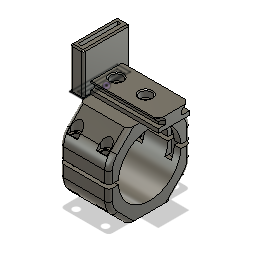
OBS-D-003 v10 (Autodesk Fusion 360 design; units mm, degrees)
Autodesk Fusion 360 part; units mm, degrees
sketch "Skizze1" plane through (0, 0, 0) normal (1, 0, 0) x (0, 0, -1)
  line L0 (-8, 5.2) -> (-6.05, 3.25)
  line L1 (-6.05, 3.25) -> (-6.05, 2)
  line L2 (6.05, 2) -> (6.05, 3.25)
  line L3 (6.05, 3.25) -> (8, 5.2)
  line L4 (8, 5.2) -> (8, 6.5)
  line L5 (8, 6.5) -> (-8, 6.5)
  line L6 (-8, 6.5) -> (-8, 5.2)
  line L7 (-6.05, 2) -> (-8, 2)
  line L8 (-8, 2) -> (-8, 0)
  line L9 (-8, 0) -> (8, 0)
  line L10 (8, 0) -> (8, 2)
  line L11 (8, 2) -> (6.05, 2)
  line L12 (0, 6.5) -> (0, 0) construction
  dimension "d5" = 16
  dimension "d6" = 1.3
  dimension "d8" = 2
  dimension "d26" = 12.1
  dimension "d27" = 4.5
  dimension "d28" = 135
  constraint vertical L1
  constraint perpendicular L2 L5
  constraint perpendicular L5 L6
  constraint vertical L4
  constraint perpendicular L1 L7
  constraint perpendicular L7 L8
  constraint perpendicular L8 L9
  constraint perpendicular L7 L10
  constraint perpendicular L2 L11
  constraint collinear L4 L10
  constraint collinear L6 L8
  constraint midpoint L5 L12.start
  constraint midpoint L9 L12.end
  constraint symmetric L0.start L3.end L12
  constraint symmetric L0.end L2.end L12
  constraint midpoint L12.end L9
  constraint collinear L7 L11
  measures "d5" distance of L4.end L5.end
  measures "d6" distance of L0.start L5.end
  measures "d8" distance of L7 L9
  measures "d26" distance of L1 L2
  measures "d27" distance of L5 L7
  measures "d28" angle of L0 L6
extrude "Extrusion1" add sketch "Skizze1" along normal blind 34.4 makes body 1
sketch "Skizze7" plane through (0, 0, 0) normal (0, 1, 0) x (1, 0, 0)
  line L0 (0, -12) -> (-6.6, -12)
  line L1 (-6.6, -12) -> (-6.6, 12)
  line L2 (-6.6, 12) -> (0, 12)
  line L3 (0, 12) -> (0, -12)
  line L4 (-0.8, -10) -> (-4.6, -10)
  line L5 (-4.6, -10) -> (-4.6, 10)
  line L6 (-4.6, 10) -> (-0.8, 10)
  line L7 (-0.8, 10) -> (-0.8, -10)
  line L8 (0, 0) -> (-0.8, 0) construction
  line L9 (-2.7, -10) -> (-2.7, 10)
  dimension "d82" = 24
  dimension "d83" = 0.8
  dimension "d84" = 2
  dimension "d85" = 3.8
  dimension "d86" = 20
  constraint horizontal L0
  constraint vertical L1
  constraint horizontal L2
  constraint vertical L3
  constraint midpoint L8.start L3
  constraint horizontal L4
  constraint vertical L5
  constraint horizontal L6
  constraint vertical L7
  constraint coincident L8.start origin
  constraint midpoint L7 L8.end
  constraint horizontal L8
  constraint midpoint L4 L9.start
  constraint midpoint L6 L9.end
  measures "d82" distance of L0.start L2.end
  measures "d83" distance of L3 L7
  measures "d84" distance of L1 L5
  measures "d85" distance of L5 L7
  measures "d86" distance of L4.end L5.end
extrude "Extrusion17" add sketch "Skizze7" along normal blind 21.2 bodies 1
extrude "Extrusion18" add sketch "Skizze7" along normal blind 9.7 contours L4 L6 L7 L9 | L4 L5 L6 L9 bodies 1
extrude "Extrusion19" add sketch "Skizze7" against normal blind 1.5 from surface at 21.2 contours L4 L6 L7 L9 bodies 1
sketch "Skizze3" plane through (0, 0, 0) normal (1, 0, 0) x (0, 0, -1)
  circle A0 centre (-2.9687, -21) radius 16
  line L0 (18, -20) -> (18, 0)
  line L1 (18, 0) -> (-23.9374, 0)
  line L2 (-23.9374, 0) -> (-23.9374, -20)
  line L3 (13, -20) -> (-18.9374, -20) construction
  line L4 (13, -20) -> (18, -20)
  line L5 (-18.9374, -20) -> (-23.9374, -20)
  line L6 (13, -22) -> (-18.9374, -22) construction
  line L7 (13, -22) -> (18, -22)
  line L8 (18, -22) -> (18, -42)
  line L9 (18, -42) -> (-23.9374, -42)
  line L10 (-23.9374, -42) -> (-23.9374, -22)
  line L11 (-23.9374, -22) -> (-18.9374, -22)
  line L12 (-2.9687, -21) -> (-2.9687, -5) construction
  line L13 (-2.9687, -37) -> (-2.9687, -21) construction
  dimension "d29" = 32
  dimension "d30" = 5
  dimension "d31" = 5
  dimension "d32" = 18
  dimension "d33" = 1
  dimension "d34" = 1
  dimension "d35" = 5
  dimension "d37" = 5
  constraint coincident A0 L3.start
  constraint coincident A0 L3.end
  constraint horizontal L3
  constraint horizontal L4
  constraint horizontal L5
  constraint vertical L0
  constraint coincident A0 L6.start
  constraint coincident A0 L6.end
  constraint horizontal L6
  constraint perpendicular L0 L7
  constraint perpendicular L10 L11
  constraint coincident A0.centre L12.start
  constraint coincident A0 L12.end
  constraint vertical L12
  constraint horizontal L1
  constraint vertical L2
  constraint vertical L8
  constraint horizontal L9
  constraint vertical L10
  constraint collinear L2 L10
  constraint collinear L0 L8
  constraint coincident A0 L13.start
  constraint perpendicular L6 L13
  constraint coincident origin L1
  measures "d29" diameter of A0
  measures "d30" distance of L0.start L3.start
  measures "d31" distance of L2.end L3.end
  measures "d32" distance of origin L0
  measures "d33" distance of A0.centre L3
  measures "d34" distance of A0.centre L6
  measures "d35" vertical distance of origin L12.end
  measures "d37" distance of L9 L13.start
extrude "Extrusion6" add sketch "Skizze3" along normal blind 25 separate body contours A0 L0 L1 L2 L4 L5 | A0 L7 L8 L9 L10 L11 makes body 2 at (8.3333, -6.3069, 9.3023) makes body 3 at (16.6667, -33.2963, -7.2686)
chamfer "Fase1" distance 10 angle 45 3 edges at (12.5, 0, 23.9374) (12.5, -42, -18) (12.5, -42, 23.9374) on bodies 2 3
chamfer "Fase2" distance 10 angle 45 1 edges at (12.5, 0, -18) on bodies 2
fillet "Abrundung1" radius 10 4 edges at (12.5, -10, 23.9374) (12.5, -10, -18) (12.5, -32, 23.9374) (12.5, -32, -18) on bodies 2 3
ref_plane "Arbeitsebene1" through (0, -9, 0) normal (0, 1, 0) x (0, 0, 1)
sketch "Skizze4" plane through (0, -9, 0) normal (0, 1, 0) x (1, 0, 0)
  line L0 (0, -2.9687) -> (5, -2.9687) construction
  line L1 (3.4, 14.6313) -> (3.4, -20.5687)
  arc A0 (3.4, -20.5687) -> (6.6, -20.5687) centre (5, -20.5687) ccw
  line L2 (6.6, -20.5687) -> (6.6, 14.6313)
  arc A1 (6.6, 14.6313) -> (3.4, 14.6313) centre (5, 14.6313) ccw
  line L3 (5, 14.6313) -> (5, -20.5687) construction
  arc A2 (6.6, -20.5687) -> (3.4, -20.5687) centre (5, -20.5687) ccw
  arc A3 (3.4, 14.6313) -> (6.6, 14.6313) centre (5, 14.6313) ccw
  line L4 (7.75, 14.6313) -> (7.75, 22.6313)
  arc A4 (7.75, 22.6313) -> (2.25, 22.6313) centre (5, 22.6313) ccw
  line L5 (2.25, 22.6313) -> (2.25, 14.6313)
  arc A5 (2.25, 14.6313) -> (7.75, 14.6313) centre (5, 14.6313) ccw
  line L6 (5, 14.6313) -> (5, 22.6313) construction
  line L7 (2.25, -20.5687) -> (2.25, -28.5687)
  arc A6 (2.25, -28.5687) -> (7.75, -28.5687) centre (5, -28.5687) ccw
  line L8 (7.75, -28.5687) -> (7.75, -20.5687)
  arc A7 (7.75, -20.5687) -> (2.25, -20.5687) centre (5, -20.5687) ccw
  line L9 (5, -20.5687) -> (5, -28.5687) construction
  line L10 (12.5, 16.976) -> (12.5, -37.3443) construction
  arc A8 (22.75, 22.6313) -> (17.25, 22.6313) centre (20, 22.6313) ccw
  line L11 (17.25, 14.6313) -> (17.25, 22.6313)
  line L12 (18.4, -20.5687) -> (18.4, 14.6313)
  arc A9 (21.6, -20.5687) -> (18.4, -20.5687) centre (20, -20.5687) ccw
  line L13 (17.25, -28.5687) -> (17.25, -20.5687)
  arc A10 (21.6, 14.6313) -> (18.4, 14.6313) centre (20, 14.6313) ccw
  arc A11 (17.25, -28.5687) -> (22.75, -28.5687) centre (20, -28.5687) ccw
  arc A12 (22.75, -20.5687) -> (17.25, -20.5687) centre (20, -20.5687) ccw
  line L14 (22.75, 22.6313) -> (22.75, 14.6313)
  line L15 (20, 14.6313) -> (20, -20.5687) construction
  arc A13 (18.4, -20.5687) -> (21.6, -20.5687) centre (20, -20.5687) ccw
  line L16 (20, -20.5687) -> (20, -28.5687) construction
  line L17 (22.75, -20.5687) -> (22.75, -28.5687)
  line L18 (20, 14.6313) -> (20, 22.6313) construction
  arc A14 (18.4, 14.6313) -> (21.6, 14.6313) centre (20, 14.6313) ccw
  line L19 (21.6, 14.6313) -> (21.6, -20.5687)
  arc A15 (17.25, 14.6313) -> (22.75, 14.6313) centre (20, 14.6313) ccw
  line L20 (2.25, 16.2313) -> (7.75, 16.2313)
  line L21 (6.6, 16.2313) -> (6.6, 13.0313)
  line L22 (7.2366, 13.0313) -> (2.7634, 13.0313)
  line L23 (3.4, 13.0313) -> (3.4, 16.2313)
  line L24 (17.25, 16.2313) -> (22.75, 16.2313)
  line L25 (21.6, 16.2313) -> (21.6, 13.0313)
  line L26 (22.2366, 13.0313) -> (17.7634, 13.0313)
  line L27 (18.4, 13.0313) -> (18.4, 16.2313)
  line L28 (2.7634, -18.9687) -> (7.2366, -18.9687)
  line L29 (6.6, -18.9687) -> (6.6, -22.1687)
  line L30 (7.75, -22.1687) -> (2.25, -22.1687)
  line L31 (3.4, -22.1687) -> (3.4, -18.9687)
  line L32 (17.7634, -18.9687) -> (22.2366, -18.9687)
  line L33 (21.6, -18.9687) -> (21.6, -22.1687)
  line L34 (22.75, -22.1687) -> (17.25, -22.1687)
  line L35 (18.4, -22.1687) -> (18.4, -18.9687)
  point P0 (0, -2.9687)
  point P1 (5, -2.9687)
  point P2 (5, -18.9687)
  point P3 (5, 13.0313)
  point P4 (20, -2.9687)
  point P5 (20, 13.0313)
  point P6 (20, -2.9687)
  point P7 (20, -18.9687)
  dimension "d43" = 5
  dimension "d44" = 1.6
  dimension "d45" = 32
  dimension "d46" = 5.5
  dimension "d47" = 5.5
  dimension "d48" = 8
  dimension "d49" = 8
  dimension "d59" = 12.5
  constraint horizontal L0
  constraint tangent L1 A0
  constraint tangent A0 L2
  constraint parallel L1 L2
  constraint tangent L2 A1
  constraint tangent L1 A1
  constraint perpendicular L0 L3
  constraint coincident P1 L0.end
  constraint midpoint L3 P1
  constraint tangent L1 A2
  constraint tangent L2 A3
  constraint midpoint A2 P2
  constraint midpoint A3 P3
  constraint tangent L4 A4
  constraint tangent A4 L5
  constraint parallel L4 L5
  constraint tangent L5 A5
  constraint tangent L4 A5
  constraint parallel L3 L6
  constraint coincident A1.centre L3.start
  constraint tangent L7 A6
  constraint tangent A6 L8
  constraint parallel L7 L8
  constraint tangent L8 A7
  constraint tangent L7 A7
  constraint parallel L3 L9
  constraint coincident A0.centre L3.end
  constraint vertical L10
  constraint symmetric P1 L10 P6
  constraint symmetric L1.start L10 A10.start
  constraint symmetric L1.end L10 A9.start
  constraint symmetric A0.end L10 L12.start
  constraint symmetric L2.end L10 L12.end
  constraint symmetric A0 L10 A13
  constraint symmetric A1 L10 A10
  constraint symmetric A2 L10 A9
  constraint symmetric A3 L10 A14
  constraint symmetric P2 L10 P7
  constraint symmetric P3 L10 P5
  constraint symmetric L4.start L10 L11.start
  constraint symmetric L4.end L10 A8.end
  constraint symmetric A4.end L10 A8.start
  constraint symmetric L5.end L10 L14.end
  constraint symmetric A4 L10 A8
  constraint symmetric A5 L10 A15
  constraint symmetric L7.start L10 A12.start
  constraint symmetric L7.end L10 A11.end
  constraint symmetric A6.end L10 L13.start
  constraint symmetric L8.end L10 L13.end
  constraint symmetric A6 L10 A11
  constraint symmetric A7 L10 A12
  constraint horizontal L20
  constraint vertical L21
  constraint horizontal L22
  constraint vertical L23
  constraint horizontal L24
  constraint vertical L25
  constraint horizontal L26
  constraint vertical L27
  constraint horizontal L28
  constraint vertical L29
  constraint horizontal L30
  constraint vertical L31
  constraint horizontal L32
  constraint vertical L33
  constraint horizontal L34
  constraint vertical L35
  constraint tangent A0 L29
  constraint tangent A2 L28
  constraint tangent A2 L31
  constraint tangent A0 L30
  constraint tangent A13 L33
  constraint tangent A9 L32
  constraint tangent A13 L35
  constraint tangent A13 L34
  constraint tangent A10 L25
  constraint tangent A10 L27
  constraint tangent A10 L24
  constraint tangent A14 L26
  constraint tangent A3 L22
  constraint tangent A3 L21
  constraint tangent A1 L23
  constraint tangent A1 L20
  constraint coincident L4 L20.end
  constraint coincident L21.start L20
  constraint coincident A5 L22.start
  constraint coincident L21.end L22
  constraint coincident A5 L22.end
  constraint coincident L23.start L22
  constraint coincident L5 L20.start
  constraint coincident L23.end L20
  constraint coincident L11 L24.start
  constraint coincident L27.end L24
  constraint coincident A15 L26.end
  constraint coincident L27.start L26
  constraint coincident A15 L26.start
  constraint coincident L25.end L26
  constraint coincident L14 L24.end
  constraint coincident L25.start L24
  constraint coincident A12 L32.start
  constraint coincident L35.end L32
  constraint coincident A12 L32.end
  constraint coincident L33.start L32
  constraint coincident L33.end L34
  constraint coincident L35.start L34
  constraint coincident A7 L28.end
  constraint coincident L29.start L28
  constraint coincident L29.end L30
  constraint coincident L31.start L30
  constraint coincident A7 L28.start
  constraint coincident L31.end L28
  constraint coincident P0 L0
  constraint coincident P0 L0.start
  measures "d43" distance of P0 P1
  measures "d44" radius of A0
  measures "d45" distance of P2 P3
  measures "d46" distance of L4 L5
  measures "d47" distance of L7 L8
  measures "d48" distance of A1.centre A4.centre
  measures "d49" distance of A0.centre A6.centre
  measures "d59" distance of P0 L10
extrude "Extrusion7" cut sketch "Skizze4" along normal up to surface (9 mm away) contours L1 A3 L22 L23 | A1 L20 L23 | A1 A3 | L1 L5 A5 L20 L22 L23 | L1 L2 A5 L22 | L1 A5 L22 | A1 L20 L21 | L4 A4 L5 L20 | L2 A3 L21 L22 | L2 L4 A5 L20 L21 L22 | L2 A5 L22 | L1 L2 A7 L28 | L1 A7 L28 | L1 A2 L28 L31 | L1 L7 A7 L28 L30 L31 | L2 A7 L28 | A0 A2 | A0 L30 L31 | L2 A2 L28 L29 | L2 L8 A7 L28 L29 L30 | A0 L29 L30 | L7 A6 L8 L30 | A8 L11 L14 L24 | L14 L19 A15 L24 L25 L26 | L11 L12 A15 L24 L26 L27 | A10 L24 L25 | A10 L24 L27 | L19 A15 L26 | A10 A14 | A14 L19 L25 L26 | L12 A15 L26 | L12 A14 L26 L27 | L12 L19 A15 L26 | L12 A12 L19 L32 | A12 L19 L32 | L12 A12 L32 | A12 L17 L19 L32 L33 L34 | A9 L19 L32 L33 | L12 A9 L32 L35 | L12 L13 A12 L32 L34 L35 | A9 A13 | A13 L33 L34 | A13 L34 L35 | L13 A11 L17 L34 bodies 2
extrude "Extrusion8" cut sketch "Skizze4" along normal blind -19 and the other way blind 3 contours L1 A3 L22 L23 | A1 A3 | L1 L2 A5 L22 | L2 A3 L21 L22 | L1 L2 A5 A7 | L1 L2 A7 L28 | L1 A2 L28 L31 | A0 A2 | L2 A2 L28 L29 | A10 A14 | A14 L19 L25 L26 | L12 A14 L26 L27 | L12 L19 A15 L26 | L12 A12 L19 A15 | L12 A12 L19 L32 | A9 L19 L32 L33 | L12 A9 L32 L35 | A9 A13 bodies 2 3
extrude "Extrusion9" cut sketch "Skizze4" against normal blind 37 contours A1 A3 | A0 A2 | A10 A14 | A9 A13 bodies 2 3
extrude "Extrusion13" cut sketch "Skizze4" against normal blind 0.3 contours L1 L5 A5 L20 L22 L23 | L2 L4 A5 L20 L21 L22 | L1 L7 A7 L28 L30 L31 | L2 L8 A7 L28 L29 L30 | L14 L19 A15 L24 L25 L26 | L11 L12 A15 L24 L26 L27 | A12 L17 L19 L32 L33 L34 | L12 L13 A12 L32 L34 L35 bodies 2
extrude "Extrusion14" cut sketch "Skizze4" against normal blind 0.6 contours L1 A3 L22 L23 | A1 L20 L23 | A1 L20 L21 | L2 A3 L21 L22 | L1 A2 L28 L31 | A0 L30 L31 | L2 A2 L28 L29 | A0 L29 L30 | A10 L24 L25 | A10 L24 L27 | A14 L19 L25 L26 | L12 A14 L26 L27 | A9 L19 L32 L33 | L12 A9 L32 L35 | A13 L33 L34 | A13 L34 L35 bodies 2
ref_plane "Arbeitsebene2" through (0, -33, 0) normal (0, 1, 0) x (0, 0, 1)
sketch "Skizze5" plane through (0, -33, 0) normal (0, 1, 0) x (1, 0, 0)
  arc A0 (21.6, 14.6313) -> (18.4, 14.6313) centre (20, 14.6313) ccw
  arc A1 (6.6, 14.6313) -> (3.4, 14.6313) centre (5, 14.6313) ccw
  arc A2 (3.4, -20.5687) -> (6.6, -20.5687) centre (5, -20.5687) ccw
  arc A3 (18.4, -20.5687) -> (21.6, -20.5687) centre (20, -20.5687) ccw
  line L0 (2.2, 13.0147) -> (5, 11.3981)
  line L1 (5, 11.3981) -> (7.8, 13.0147)
  line L2 (7.8, 13.0147) -> (7.8, 16.2479)
  line L3 (7.8, 16.2479) -> (5, 17.8644)
  line L4 (5, 17.8644) -> (2.2, 16.2479)
  line L5 (2.2, 16.2479) -> (2.2, 13.0147)
  line L6 (2.2, -22.1853) -> (5, -23.8019)
  line L7 (5, -23.8019) -> (7.8, -22.1853)
  line L8 (7.8, -22.1853) -> (7.8, -18.9521)
  line L9 (7.8, -18.9521) -> (5, -17.3356)
  line L10 (5, -17.3356) -> (2.2, -18.9521)
  line L11 (2.2, -18.9521) -> (2.2, -22.1853)
  line L12 (17.2, -22.1853) -> (20, -23.8019)
  line L13 (20, -23.8019) -> (22.8, -22.1853)
  line L14 (22.8, -22.1853) -> (22.8, -18.9521)
  line L15 (22.8, -18.9521) -> (20, -17.3356)
  line L16 (20, -17.3356) -> (17.2, -18.9521)
  line L17 (17.2, -18.9521) -> (17.2, -22.1853)
  line L18 (17.2, 13.0147) -> (20, 11.3981)
  line L19 (20, 11.3981) -> (22.8, 13.0147)
  line L20 (22.8, 13.0147) -> (22.8, 16.2479)
  line L21 (22.8, 16.2479) -> (20, 17.8644)
  line L22 (20, 17.8644) -> (17.2, 16.2479)
  line L23 (17.2, 16.2479) -> (17.2, 13.0147)
  arc A4 (21.6, -20.5687) -> (18.4, -20.5687) centre (20, -20.5687) ccw
  arc A5 (6.6, -20.5687) -> (3.4, -20.5687) centre (5, -20.5687) ccw
  arc A6 (3.4, 14.6313) -> (6.6, 14.6313) centre (5, 14.6313) ccw
  arc A7 (18.4, 14.6313) -> (21.6, 14.6313) centre (20, 14.6313) ccw
  line L24 (2.2, -22.1853) -> (7.8, -22.1853)
  line L25 (7.8, -18.9521) -> (2.2, -18.9521)
  line L26 (17.2, -22.1853) -> (22.8, -22.1853)
  line L27 (22.8, -18.9521) -> (17.2, -18.9521)
  line L28 (7.8, 13.0147) -> (2.2, 13.0147)
  line L29 (2.2, 16.2479) -> (7.8, 16.2479)
  line L30 (17.2, 16.2479) -> (22.8, 16.2479)
  line L31 (22.8, 13.0147) -> (17.2, 13.0147)
  line L32 (21.6, 13.0147) -> (21.6, 10.2479)
  line L33 (18.4, 13.0147) -> (18.4, 16.2479)
  line L34 (3.4, 13.0147) -> (3.4, 16.2479)
  line L35 (6.6, 16.2479) -> (6.6, 13.0147)
  line L36 (3.4, -22.1853) -> (3.4, -18.9521)
  line L37 (6.6, -18.9521) -> (6.6, -22.1853)
  line L38 (18.4, -22.1853) -> (18.4, -18.9521)
  line L39 (21.6, -22.1853) -> (21.6, -18.9521)
  point P0 (5, 14.6313)
  point P1 (20, 14.6313)
  point P2 (20, -20.5687)
  point P3 (5, -20.5687)
  point P4 (5, 14.6313)
  point P5 (5, -20.5687)
  point P6 (20, -20.5687)
  point P7 (20, 14.6313)
  dimension "d61" = 5.6
  constraint coincident P4 P0
  constraint coincident P5 P3
  constraint coincident P6 P2
  constraint coincident P7 P1
  constraint equal L2 L23
  constraint equal L2 L8
  constraint equal L8 L17
  constraint vertical L5
  constraint vertical L23
  constraint vertical L17
  constraint vertical L11
  constraint coincident L31 L32.start
  constraint perpendicular L31 L32
  constraint coincident L31 L33.start
  constraint coincident L30 L33.end
  constraint perpendicular L30 L33
  constraint coincident L28 L34.start
  constraint coincident L29 L34.end
  constraint perpendicular L29 L34
  constraint coincident L29 L35.start
  constraint coincident L28 L35.end
  constraint perpendicular L28 L35
  constraint tangent A7 L32
  constraint tangent A7 L33
  constraint tangent A6 L35
  constraint tangent A6 L34
  constraint coincident L24 L36.start
  constraint coincident L25 L36.end
  constraint perpendicular L25 L36
  constraint coincident L25 L37.start
  constraint coincident L24 L37.end
  constraint perpendicular L24 L37
  constraint coincident L26 L38.start
  constraint coincident L27 L38.end
  constraint perpendicular L27 L38
  constraint coincident L26 L39.start
  constraint coincident L27 L39.end
  constraint perpendicular L27 L39
  constraint tangent A2 L36
  constraint tangent A2 L37
  constraint tangent A3 L38
  constraint tangent A3 L39
  measures "d61" distance of L2 L5
extrude "Extrusion10" cut sketch "Skizze5" against normal blind 17 contours A0 A7 | L20 L30 L31 L33 | L23 L30 L31 L33 | L18 L19 L31 L32 | L21 L22 L30 | L19 L31 L32 | A1 A6 | A6 L28 L34 L35 | A1 L29 L34 L35 | L2 L28 L29 L35 | L5 L28 L29 L34 | L3 L4 L29 | L0 L1 L28 | A2 A5 | A5 L25 L36 L37 | A2 L24 L36 L37 | L11 L24 L25 L36 | L8 L24 L25 L37 | L6 L7 L24 | L9 L10 L25 | A3 A4 | A4 L27 L38 L39 | A3 L26 L38 L39 | L17 L26 L27 L38 | L14 L26 L27 L39 | L12 L13 L26 | L15 L16 L27 bodies 3
extrude "Extrusion11" cut sketch "Skizze5" along normal blind 0.3 contours L20 L30 L31 L33 | L23 L30 L31 L33 | L2 L28 L29 L35 | L5 L28 L29 L34 | L11 L24 L25 L36 | L8 L24 L25 L37 | L17 L26 L27 L38 | L14 L26 L27 L39 bodies 3
extrude "Extrusion12" cut sketch "Skizze5" along normal blind 0.6 contours L20 L30 L31 L33 | A6 L28 L34 L35 | A1 L29 L34 L35 | A5 L25 L36 L37 | A2 L24 L36 L37 | A4 L27 L38 L39 | A3 L26 L38 L39 bodies 3
sketch "Skizze6" plane through (0, 0, 0) normal (0, 1, 0) x (1, 0, 0)
  line L0 (0, 0) -> (0.2903, 0)
  line L1 (0.2903, 0) -> (23.3187, 0) construction
  circle A0 centre (5, 0) radius 1.6
  circle A1 centre (20, 0) radius 1.6
  line L2 (22.8, 1.6166) -> (20, 3.2332)
  line L3 (20, 3.2332) -> (17.2, 1.6166)
  line L4 (17.2, 1.6166) -> (17.2, -1.6166)
  line L5 (17.2, -1.6166) -> (20, -3.2332)
  line L6 (20, -3.2332) -> (22.8, -1.6166)
  line L7 (22.8, -1.6166) -> (22.8, 1.6166)
  line L8 (7.8, 1.6166) -> (5, 3.2332)
  line L9 (5, 3.2332) -> (2.2, 1.6166)
  line L10 (2.2, 1.6166) -> (2.2, -1.6166)
  line L11 (2.2, -1.6166) -> (5, -3.2332)
  line L12 (5, -3.2332) -> (7.8, -1.6166)
  line L13 (7.8, -1.6166) -> (7.8, 1.6166)
  point P0 (20, 0)
  point P1 (5, 0)
  dimension "d72" = 20
  dimension "d73" = 5
  dimension "d74" = 3.2
  dimension "d75" = 5.6
  constraint coincident L0.start origin
  constraint horizontal L0
  constraint parallel L0 L1
  constraint coincident L1 P1
  constraint coincident L1 P0
  constraint equal A0 A1
  constraint coincident P0 A1.centre
  constraint coincident P1 A0.centre
  constraint equal L4 L13
  constraint vertical L13
  constraint vertical L4
  measures "d72" distance of L0.start A1.centre
  measures "d73" distance of L0.start P1
  measures "d74" diameter of A0
  measures "d75" distance of L4 L7
extrude "Extrusion15" cut sketch "Skizze6" against normal blind 11 contours A0 | A1 bodies 2
extrude "Extrusion16" cut sketch "Skizze6" along normal blind -12.5 and the other way blind 2 bodies 2
sketch "Skizze9" plane through (0, 6.5, 0) normal (0, 1, 0) x (-1, 0, 0)
  line L0 (0, -8) -> (0, 8)
  line L1 (0, 8) -> (-34.4, 8)
  line L2 (-34.4, 8) -> (-34.4, -8)
  line L3 (-34.4, -8) -> (0, -8)
  circle A0 centre (-5, 0) radius 1.6
  circle A1 centre (-20, 0) radius 1.6
  circle A2 centre (-20, 0) radius 3
  circle A3 centre (-5, 0) radius 3
  dimension "d94" = 6
  constraint concentric A1 A2
  constraint concentric A0 A3
  constraint equal A2 A3
  measures "d94" diameter of A2
extrude "Extrusion20" cut sketch "Skizze9" against normal blind 4 contours A2 | A3 bodies 1
extrude "Extrusion21" cut sketch "Skizze9" against normal blind 11 contours A0 | A1 bodies 1
fillet "Abrundung2" radius 2 24 edges at (0, -3.5355, 17.473) (0, -10.3153, 23.1762) (0, -17.0711, 23.9374) (25, -17.0711, 23.9374) (25, -10.3153, 23.1762) (25, -3.5355, 17.473) (0, -17.0711, -18) (0, -10.3153, -17.2388) (0, -3.5355, -11.5355) (25, -3.5355, -11.5355) (25, -10.3153, -17.2388) (25, -17.0711, -18) (25, -38.4645, -11.5355) (25, -31.6847, -17.2388) (25, -24.9289, -18) (0, -24.9289, -18) (0, -31.6847, -17.2388) (0, -38.4645, -11.5355) (25, -24.9289, 23.9374) (25, -31.6847, 23.1762) (25, -38.4645, 17.473) (0, -38.4645, 17.473) (0, -31.6847, 23.1762) (0, -24.9289, 23.9374) on bodies 2 3
fillet "Abrundung3" radius 1 4 edges at (0, 10.6, -12) (-6.6, 10.6, -12) (0, 10.6, 12) (-6.6, 10.6, 12) on bodies 1
chamfer "Fase3" distance 0.5 angle 45 9 edges at (0, 0, -9.5) (-0.2929, 0, -11.7071) (-3.3, 0, -12) (-6.3071, 0, -11.7071) (-6.6, 0, 0) (-6.3071, 0, 11.7071) (-3.3, 0, 12) (-0.2929, 0, 11.7071) (0, 0, 9.5) on bodies 1
chamfer "Fase4" distance 2 angle 45 6 edges at (34.4, 2.625, -6.05) (34.4, 2.625, 6.05) (34.4, 5.85, 8) (34.4, 5.85, -8) (34.4, 4.225, 7.025) (34.4, 4.225, -7.025) on bodies 1
extrude "Extrusion22" cut sketch "Skizze9" against normal blind 0.5 contours L0 L1 L2 L3 bodies 1
chamfer "Fase5" distance 0.7 angle 45 8 edges at (-3.3, 21.2, 12) (-6.3071, 21.2, 11.7071) (-6.6, 21.2, 0) (-6.3071, 21.2, -11.7071) (-3.3, 21.2, -12) (-0.2929, 21.2, -11.7071) (0, 21.2, 0) (-0.2929, 21.2, 11.7071) on bodies 1
chamfer "Fase6" distance 0.5 angle 45 2 edges at (22.797, 6, -1.0848) (7.797, 6, -1.0848) on bodies 1
equation "d72 = 25 mm - 5 mm"
equation "d87 = 9.7 mm + 10 mm + 1.5 mm"
